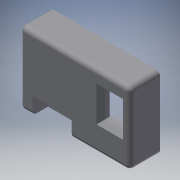
# Autodesk Inventor part: HapticFeedbackCase
Saved by Autodesk Inventor 2016 (Build 200138000, 138)
## iProperties
Created: 2015-09-22
Part Number: HapticFeedbackCase
Material: Generic
Document SubType Name: Modeling
Designer: Jake
Density: 1 g/cm^3
Appearance: Default
Author: Jake
Autodesk Inventor part; units mm, degrees
ref_plane "YZ Plane" through (0, 0, 0) normal (1, 0, 0) x (0, 1, 0)
ref_plane "XZ Plane" through (0, 0, 0) normal (0, 1, 0) x (-1, 0, 0)
ref_plane "XY Plane" through (0, 0, 0) normal (0, 0, 1) x (1, 0, 0)
sketch "Sketch2" plane through (0, 0, 0) normal (0, 0, 1) x (1, 0, 0)
  line L0 (0, 0) -> (26.67, 0)
  line L1 (26.67, 0) -> (26.67, 15.748)
  line L2 (26.67, 15.748) -> (0, 15.748)
  line L3 (0, 15.748) -> (0, 0)
  dimension "d4" = 26.67
  dimension "d5" = 15.748
  dimension "d6" = 26.67
  constraints: 8 end point, 2 perpendicular, 1 horizontal
  measures "d4" distance of L0.start L0.end
  measures "d5" distance of L0.end L1.end
  measures "d6" distance of L1.end L2.end
sketch "Sketch3" plane through (0, 0, 0) normal (0, 0, 1) x (1, 0, 0)
  line L0 (0, -2.54) -> (29.21, -2.54)
  line L1 (29.21, -2.54) -> (29.21, 15.748)
  line L2 (29.21, 15.748) -> (29.21, 18.288)
  line L3 (29.21, 18.288) -> (-2.54, 18.288)
  line L4 (-2.54, 18.288) -> (-2.54, -2.54)
  line L5 (-2.54, -2.54) -> (0, -2.54)
  line L6 (-2.54, -2.54) -> (29.21, -2.54)
  line L7 (29.21, 18.288) -> (-2.54, 18.288)
  line L8 (-2.54, 18.288) -> (-2.54, -2.54)
  point P0 (0, 0)
  dimension "d7" = 2.54
  dimension "d8" = 29.21
  dimension "d9" = 18.288
  dimension "d10" = 2.54
  dimension "d11" = 31.75
  constraints: 18 end point, 5 perpendicular, 2 point on line, 1 horizontal, 1 parallel
  measures "d7" distance of point (0, 0) L0.start
  measures "d8" distance of L0.start L0.end
  measures "d9" distance of L0.end L1.end
  measures "d10" distance of L1.end L2.end
  measures "d11" distance of L2.end L3.end
extrude "Extrusion1" add sketch "Sketch3" along normal blind 5.842
extrude "Extrusion2" cut sketch "Sketch2" along normal blind 3.302
sketch "Sketch4" plane through (0, 0, 5.842) normal (0, 0, 1) x (1, 0, 0)
  line L0 (0, 15.748) -> (0, 0) projected
  line L1 (10.16, 0.254) -> (10.16, -2.54)
  line L2 (-2.54, -2.54) -> (29.21, -2.54) projected
  line L3 (0, -2.54) -> (0, 0)
  line L4 (0, -2.54) -> (10.16, -2.54)
  line L5 (0, 0) -> (0, 2.54)
  line L6 (0, 2.54) -> (10.16, 2.54)
  line L7 (10.16, 2.54) -> (10.16, 0.254)
  line L8 (10.16, -2.54) -> (10.16, 0.254)
  dimension "d18" = 2.54
  dimension "d19" = 10.16
  constraints: 14 end point, 3 perpendicular, 3 point on line, 1 collinear, 1 parallel
  measures "d18" distance of L0.end L5.end
  measures "d19" distance of L5.end L6.end
extrude "Extrusion3" cut sketch "Sketch4" against normal blind 3.302
sketch "Sketch5" plane through (0, 0, 5.842) normal (0, 0, 1) x (1, 0, 0)
  line L0 (29.21, 18.288) -> (-2.54, 18.288) projected
  line L1 (0, 18.288) -> (29.21, 18.288)
  line L2 (29.21, 18.288) -> (29.21, 0)
  line L3 (29.21, 18.288) -> (20.828, 18.288)
  line L4 (29.21, 18.288) -> (25.4, 18.288)
  line L5 (25.4, 18.288) -> (25.4, 15.748)
  line L6 (20.828, 18.288) -> (20.828, 13.462)
  line L7 (20.828, 13.462) -> (20.828, 1.524)
  line L8 (25.4, 18.288) -> (25.4, 13.462)
  line L9 (25.4, 13.462) -> (20.828, 13.462)
  line L10 (25.4, 1.524) -> (20.828, 1.524)
  line L11 (29.21, -2.54) -> (29.21, 18.288) projected
  line L12 (29.21, 13.462) -> (25.908, 13.462)
  line L13 (25.908, 13.462) -> (25.908, 1.524)
  line L14 (25.908, 1.524) -> (25.4, 1.524)
  line L15 (25.908, 13.462) -> (25.4, 13.462)
  line L16 (20.828, 1.524) -> (25.908, 1.524)
  line L17 (25.908, 13.462) -> (25.908, 1.524)
  line L18 (20.828, 1.524) -> (25.908, 1.524)
  line L19 (20.828, 13.462) -> (20.828, 5.842)
  line L20 (20.828, 5.842) -> (25.908, 5.842)
  point P0 (0, 0)
  dimension "d22" = 8.382
  dimension "d23" = 3.81
  dimension "d24" = 2.54
  dimension "d25" = 4.826
  dimension "d26" = 11.938
  dimension "d28" = 3.302
  dimension "d80" = 7.62
  constraints: 38 end point, 7 perpendicular, 7 point on line, 3 collinear, 2 horizontal, 1 vertical
  measures "d22" distance of L0.start L3.end
  measures "d23" distance of L0.start L4.end
  measures "d24" distance of L4.end L5.end
  measures "d25" distance of L3.end L6.end
  measures "d26" distance of L6.end L7.end
  measures "d28" distance of L12.start L12.end
  measures "d80" distance of L6.end L19.end
extrude "Extrusion4" cut sketch "Sketch5" against normal blind 3.302 contours L13 L20 L7 L9 L15 | L13 L14 L10 L7 L20
move faces "Move1" translate (0, 0, -1.6002) faces at (8.89, 17.4413, 0)
move faces "Move2" translate (0, 0, -1.27) faces at (8.89, 17.4413, -1.6002)
sketch "Sketch8" plane through (29.21, -2.54, -1.6002) normal (0, 0, -1) x (-1, 0, 0)
  line L0 (31.75, 0) -> (15.875, 0)
  line L1 (19.05, 0) -> (0, 0) projected
  line L2 (31.75, 0) -> (31.75, 10.414)
  line L3 (0, 20.828) -> (31.75, 20.828) projected
  line L4 (31.75, 10.414) -> (0, 10.414)
  line L5 (0, 0) -> (0, 20.828) projected
  line L6 (15.875, 0) -> (15.875, 20.828)
  line L7 (18.415, 19.05) -> (18.415, 20.828)
  line L8 (13.335, 19.05) -> (13.335, 20.828)
  line L9 (18.415, 20.828) -> (13.335, 20.828)
  line L10 (31.75, 10.414) -> (31.75, 12.954)
  line L11 (31.75, 20.828) -> (31.75, 0) projected
  line L12 (31.75, 12.954) -> (29.21, 12.954)
  line L13 (29.21, 18.288) -> (29.21, 2.54) projected
  line L14 (29.21, 12.954) -> (29.21, 7.874)
  line L15 (29.21, 7.874) -> (31.75, 7.874)
  line L16 (31.75, 12.954) -> (31.75, 7.874)
  line L17 (0, 10.414) -> (0, 7.874)
  line L18 (0, 7.874) -> (2.54, 7.874)
  line L19 (2.54, 2.54) -> (2.54, 18.288) projected
  line L20 (2.54, 7.874) -> (2.54, 12.954)
  line L21 (2.54, 12.954) -> (0, 12.954)
  line L22 (0, 10.414) -> (0, 12.954)
  line L23 (18.415, 20.828) -> (18.415, 18.288)
  line L24 (18.415, 18.288) -> (13.335, 18.288)
  line L25 (2.54, 18.288) -> (29.21, 18.288) projected
  line L26 (13.335, 19.05) -> (13.335, 18.288)
  dimension "d36" = 15.875
  dimension "d37" = 10.414
  dimension "d40" = 2.54
  dimension "d41" = 5.08
  dimension "d42" = 2.54
  dimension "d43" = 5.08
  constraints: 40 end point, 12 point on line, 7 perpendicular, 2 collinear, 2 midpoint, 1 vertical
  measures "d36" distance of L0.start L0.end
  measures "d37" distance of L0.start L2.end
  measures "d40" distance of L2.end L10.end
  measures "d41" distance of L12.end L14.end
  measures "d42" distance of L4.end L17.end
  measures "d43" distance of L18.end L20.end
sketch "Sketch9" plane through (0, 2.54, 3.302) normal (1, 0, 0) x (0, 0, -1)
  line L0 (6.1722, -2.54) -> (6.1722, 5.334)
  line L1 (6.1722, 13.208) -> (6.1722, -2.54) projected
  line L2 (6.1722, 5.334) -> (6.1722, 7.874)
  line L3 (6.1722, 7.874) -> (4.9022, 7.874)
  line L4 (4.9022, 7.874) -> (4.9022, 2.794)
  line L5 (4.9022, 2.794) -> (6.1722, 2.794)
  point P0 (3.302, -2.54)
  dimension "d47" = 7.874
  dimension "d48" = 2.54
  dimension "d49" = 1.27
  dimension "d50" = 5.08
  constraints: 10 end point, 3 perpendicular, 2 point on line, 1 midpoint
  measures "d47" distance of L0.start L0.end
  measures "d48" distance of L0.end L2.end
  measures "d49" distance of L2.end L3.end
  measures "d50" distance of L3.end L4.end
sketch "Sketch10" plane through (0, 15.748, 3.302) normal (0, -1, 0) x (1, 0, 0)
  line L0 (0, -6.1722) -> (13.335, -6.1722)
  line L1 (13.335, -6.1722) -> (15.875, -6.1722)
  line L2 (15.875, -6.1722) -> (15.875, -4.9022)
  line L3 (15.875, -4.9022) -> (10.795, -4.9022)
  line L4 (10.795, -4.9022) -> (10.795, -6.1722)
  line L5 (26.67, -6.1722) -> (0, -6.1722) projected
  line L6 (10.795, -6.1722) -> (15.875, -6.1722)
  point P0 (0, -3.302)
  dimension "d51" = 13.335
  dimension "d52" = 2.54
  dimension "d54" = 1.27
  dimension "d55" = 5.08
  constraints: 12 end point, 2 perpendicular, 1 collinear, 1 horizontal, 1 point on line, 1 vertical
  measures "d51" distance of L0.start L0.end
  measures "d52" distance of L0.end L1.end
  measures "d54" distance of L1.end L2.end
  measures "d55" distance of L2.end L3.end
extrude "Extrusion6" add sketch "Sketch10" along normal blind 1.27
sketch "Sketch11" plane through (10.795, 15.748, -2.8702) normal (-1, 0, 0) x (0, 0, 1)
  line L0 (1.27, -1.27) -> (0, -1.27)
  line L1 (0, -1.27) -> (0, 0)
  line L2 (0, 0) -> (0, -1.27) projected
  line L3 (0, 0) -> (0, -1.27)
  line L4 (0, 0) -> (1.27, -1.27)
  point P0 (2.8702, -15.748)
  constraints: 8 end point, 2 collinear, 1 horizontal
extrude "Extrusion7" cut sketch "Sketch11" against normal blind 5.08
move faces "Move3" translate (2.286, 0, 0) faces at (10.16, 0, 4.9953)
sketch "Sketch13" plane through (0, 2.54, 3.302) normal (1, 0, 0) x (0, 0, -1)
  line L0 (0.762, -2.54) -> (-0.7986, -2.54)
  line L1 (0, 0) -> (-0.0183, -2.54)
  line L2 (-2.54, 0) -> (0, 0) projected
  line L3 (0.762, -5.08) -> (-2.54, -5.08) projected
  line L4 (-2.54, 0) -> (-2.54, -5.08)
  line L5 (-2.54, -5.08) -> (0.762, -5.08)
  line L6 (0.762, -5.08) -> (0.762, -2.54)
  point P0 (3.302, -2.54)
  constraints: 10 end point, 2 perpendicular, 1 horizontal, 1 midpoint, 1 vertical
extrude "Extrusion8" add sketch "Sketch13" along normal blind 1.016
move faces "Move4" translate (0, 0, -1.27) faces at (4.826, -0.8467, 2.54)
move faces "Move5" translate (0, 4.318, 0) faces at (22.5213, 1.524, 4.9953)
chamfer "Chamfer5" distance 1.27 angle 45 4 edges at (23.368, 5.842, 5.842) (20.828, 9.652, 5.842) (23.368, 13.462, 5.842) (25.908, 9.652, 5.842)
fillet "Fillet1" radius 1.27 9 edges at (13.335, 18.288, 5.842) (-2.54, 7.874, 5.842) (-0.762, -2.54, 5.842) (20.828, -2.54, 5.842) (29.21, 7.874, 5.842) (-2.54, 18.288, 1.4859) (29.21, 18.288, 1.4859) (29.21, -2.54, 1.4859) (-2.54, -2.54, 1.4859)
body "Solid1"
